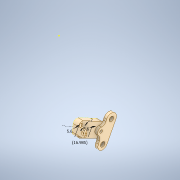
# Autodesk Inventor part: Kauri camera mount 3m bolt mount
Saved by Autodesk Inventor 2020 (Build 240168000, 168)
## iProperties
Created: 2022-04-26
Part Number: Kauri camera mount 3m bolt mount
Material: Polyethylene, High Density
Document SubType Name: Modeling
Designer: Steve3
Density: 0.952 g/cm^3
Appearance: Smooth - Off-White
Mass: 3.49117 g
Surface Area: 23.6855 cm^2
Volume: 3.6672 cm^3
Sending System: Autodesk Inventor 2020
Preprocessor: ST-DEVELOPER v18
Title: Y:\Street League\Frames\Kauri\AAA LeadFingers version 2\github files\Kauri side plate.stp
Author: Steven
Autodesk Inventor part; units mm, degrees
ref_plane "YZ Plane" through (0, 0, 0) normal (1, 0, 0) x (0, 1, 0)
ref_plane "XZ Plane" through (0, 0, 0) normal (0, 1, 0) x (-1, 0, 0)
ref_plane "XY Plane" through (0, 0, 0) normal (0, 0, 1) x (1, 0, 0)
sketch "Sketch3" plane through (0, 0, 0) normal (1, 0, 0) x (0, 1, 0)
  arc A0 (-67.955871, -10.84796) -> (-66.441009, -10.934527) centre (-66.801428, -3.943812) ccw
  line L0 (-67.955871, -10.84796) -> (-106.637607, -4.379985)
  arc A1 (-106.637607, -4.379985) -> (-109.798343, -5.963196) centre (-107.132368, -7.338906) ccw
  line L1 (-109.798343, -5.963196) -> (-127.177149, -39.641421)
  arc A2 (-127.177149, -39.641421) -> (-125.886884, -43.683106) centre (-124.511174, -41.017131) ccw
  line L2 (-125.886884, -43.683106) -> (-89.438575, -62.491345)
  arc A3 (-89.438575, -62.491345) -> (-85.311446, -54.49342) centre (-87.37501, -58.492382) ccw
  line L3 (-85.311446, -54.49342) -> (-91.002473, -51.556707)
  arc A4 (-92.937871, -45.49418) -> (-91.002473, -51.556707) centre (-88.938908, -47.557745) ccw
  line L4 (-92.937871, -45.49418) -> (-80.167513, -20.746623)
  arc A5 (-75.953198, -18.635676) -> (-80.167513, -20.746623) centre (-76.61288, -22.580903) ccw
  line L5 (-75.953198, -18.635676) -> (-69.441262, -19.724537)
  arc A6 (-69.441262, -19.724537) -> (-67.924186, -19.810989) centre (-68.286819, -12.820389) ccw
  line L6 (-67.924186, -19.810989) -> (-31.437531, -17.918268)
  arc A7 (-31.437531, -17.918268) -> (-29.900457, -17.66496) centre (-31.800164, -10.927667) ccw
  line L7 (-29.900457, -17.66496) -> (0.430435, -9.112589)
  arc A8 (1.244595, -9) -> (0.430435, -9.112589) centre (1.244595, -12) ccw
  line L8 (1.244595, -9) -> (36.324375, -9)
  arc A9 (38.324375, -11) -> (36.324375, -9) centre (36.324375, -11) ccw
  line L9 (38.324375, -11) -> (38.324375, -31.554034)
  arc A10 (38.324375, -31.554034) -> (47.324375, -31.554034) centre (42.824375, -31.554034) ccw
  line L10 (47.324375, -31.554034) -> (47.324375, -3)
  arc A11 (47.324375, -3) -> (44.324375, 0) centre (44.324375, -3) ccw
  line L11 (44.324375, 0) -> (0, 0)
  arc A12 (0, 0) -> (-0.81416, -0.112589) centre (0, -3) ccw
  line L12 (-0.81416, -0.112589) -> (-32.341858, -9.002422)
  arc A13 (-33.881146, -9.255844) -> (-32.341858, -9.002422) centre (-34.241565, -2.265129) ccw
  line L13 (-33.881146, -9.255844) -> (-66.441009, -10.934527)
  circle A14 centre (-121.30655, -39.994088) radius 1.55
  circle A15 centre (0.211343, -4.528281) radius 1.55
  circle A16 centre (42.824375, -31.554034) radius 1.55
  circle A17 centre (-105.928481, -9.742357) radius 1.55
  circle A18 centre (-101.599285, -49.7515) radius 1.55
  circle A19 centre (-31.883173, -13.503326) radius 1.55
  circle A20 centre (42.092142, -5.232233) radius 1.55
  circle A21 centre (-67.942935, -15.37073) radius 1.55
  circle A22 centre (-87.37501, -58.492382) radius 1.55
  arc A23 (-115.052095, -35.770625) -> (-113.76183, -39.81231) centre (-112.38612, -37.146335) ccw
  line L14 (-115.052095, -35.770625) -> (-105.14423, -16.570265)
  arc A24 (-100.929915, -14.459318) -> (-105.14423, -16.570265) centre (-101.589596, -18.404545) ccw
  line L15 (-100.929915, -14.459318) -> (-93.56365, -15.691031)
  arc A25 (-90.668698, -21.470538) -> (-93.56365, -15.691031) centre (-94.223331, -19.636259) ccw
  line L16 (-90.668698, -21.470538) -> (-101.165081, -41.81138)
  arc A26 (-106.553994, -43.531734) -> (-101.165081, -41.81138) centre (-104.719714, -39.9771) ccw
  line L17 (-106.553994, -43.531734) -> (-113.76183, -39.81231)
  point P0 (0, 0)
  constraints: 36 end point, 36 point on circle, 27 centre point
sketch "Sketch4" plane through (0, 0, 0) normal (1, 0, 0) x (0, 1, 0)
  circle A0 centre (-31.874031, -13.318785) radius 2.55
  circle A1 centre (-105.928481, -9.742349) radius 2.55
  circle A2 centre (-67.929027, -15.276045) radius 2.55
  arc A3 (-67.953281, -10.755052) -> (-66.596265, -10.844659) centre (-66.815732, -3.8481) ccw
  line L0 (-67.953281, -10.755052) -> (-72.057153, -10.079159)
  line L1 (-72.057153, -10.079159) -> (-106.692939, -3.305688)
  line L2 (-109.418868, -5.256805) -> (-106.692939, -3.305688)
  line L3 (-109.418868, -5.256805) -> (-109.985066, -6.360777)
  arc A4 (-109.985066, -6.360777) -> (-106.347133, -13.576326) centre (-105.536074, -8.642546) ccw
  line L4 (-106.347133, -13.576326) -> (-72.676157, -19.111461)
  line L5 (-72.676157, -19.111461) -> (-69.418112, -19.643326)
  line L6 (-69.418112, -19.643326) -> (-69.246781, -19.671535)
  arc A5 (-69.246781, -19.671535) -> (-68.163005, -19.730586) centre (-68.434471, -14.737961) ccw
  line L7 (-68.163005, -19.730586) -> (-31.193784, -17.720444)
  arc A6 (-31.193784, -17.720444) -> (-30.096328, -17.536774) centre (-31.46525, -12.727819) ccw
  line L8 (-30.096328, -17.536774) -> (-2.957928, -9.811529)
  arc A7 (-2.957928, -9.811529) -> (-2.822361, -8.911388) centre (-3.09482, -9.330633) ccw
  arc A8 (-4.999909, -2.339095) -> (-2.822361, -8.911388) centre (0.19802, -4.263787) ccw
  line L9 (-4.999909, -2.339095) -> (-5.258479, -1.511364)
  line L10 (-5.258479, -1.511364) -> (-7.95473, -1.614726)
  line L11 (-7.95473, -1.614726) -> (-29.572777, -8.030198)
  line L12 (-29.572777, -8.030198) -> (-32.007842, -8.723366)
  line L13 (-34.027372, -9.084122) -> (-32.007842, -8.723366)
  line L14 (-34.027372, -9.084122) -> (-66.596265, -10.844659)
  point P0 (0, 0)
  point P1 (-79.411985, 18.032743)
  constraints: 30 end point, 12 point on circle, 9 centre point
sketch "Sketch5" plane through (0, 0, 0) normal (1, 0, 0) x (0, 1, 0)
  line L0 (-90.668698, -21.470538) -> (-101.165081, -41.81138)
  arc A0 (-90.668698, -21.470538) -> (-93.56365, -15.691031) centre (-94.223331, -19.636259) ccw
  line L1 (-100.929915, -14.459318) -> (-93.56365, -15.691031)
  arc A1 (-100.929915, -14.459318) -> (-105.14423, -16.570265) centre (-101.589596, -18.404545) ccw
  line L2 (-115.052095, -35.770625) -> (-105.14423, -16.570265)
  arc A2 (-115.052095, -35.770625) -> (-113.76183, -39.81231) centre (-112.38612, -37.146335) ccw
  line L3 (-106.553994, -43.531734) -> (-113.76183, -39.81231)
  arc A3 (-106.553994, -43.531734) -> (-101.165081, -41.81138) centre (-104.719714, -39.9771) ccw
  line L4 (-101.253947, -41.765523) -> (-90.757564, -21.424681)
  arc A4 (-90.757564, -21.424681) -> (-93.580142, -15.789662) centre (-94.223331, -19.636259) ccw
  line L5 (-93.580142, -15.789662) -> (-100.946407, -14.557948)
  arc A5 (-100.946407, -14.557948) -> (-105.055364, -16.616122) centre (-101.589596, -18.404545) ccw
  line L6 (-105.055364, -16.616122) -> (-114.963229, -35.816482)
  arc A6 (-114.963229, -35.816482) -> (-113.715973, -39.723444) centre (-112.38612, -37.146335) ccw
  line L7 (-113.715973, -39.723444) -> (-106.508137, -43.442868)
  arc A7 (-106.508137, -43.442868) -> (-101.253947, -41.765523) centre (-104.719714, -39.9771) ccw
  point P0 (0, 0)
  dimension "d0" = 0.1
  constraints: 8 end point, 8 point on circle, 4 centre point, 7 other
  measures "d0" distance between parallel lines of L0 L4
extrude "Extrusion1" add sketch "Sketch5" along normal blind 6 contours A7 L7 A6 L6 A5 L5 A4 L4
sketch "Sketch6" plane through (0, -100.946407, -14.557948) normal (0, 0.1649204, 0.9863069) x (1, 0, 0)
  line L0 (6, 7.468532) -> (6, 0) construction
  line L1 (6, 3.734266) -> (14, 3.734266) construction
  line L2 (6, 3.734266) -> (6, 7.734266) construction
  line L3 (6, 7.734266) -> (14, 7.734266)
  line L4 (14, 7.734266) -> (14, -0.265734)
  line L5 (14, -0.265734) -> (6, -0.265734)
  line L6 (6, -0.265734) -> (6, 7.734266)
  point P0 (0, 97.163232)
  dimension "d3" = 8
  dimension "d4" = 4
  dimension "d5" = 8
  constraints: 12 end point, 2 horizontal, 2 parallel, 1 midpoint, 1 perpendicular, 1 point on line
  measures "d3" distance of L1.start L1.end
  measures "d4" distance of L1.start L2.end
  measures "d5" distance of L3.end L4.end
extrude "Extrusion2" add sketch "Sketch6" against normal blind 2
fillet "Fillet1" radius 3 2 edges at (14, -101.3734, -15.5004) (14, -93.483, -16.8198)
sketch "Sketch7" plane through (0, -101.276247, -16.530562) normal (0, -0.1649204, -0.9863069) x (-1, 0, 0)
  line L0 (-14, 4.734266) -> (-14, 2.734266)
  line L1 (-14, 2.734266) -> (-14, 4.734266) construction
  line L2 (-14, 3.734266) -> (-11.2, 3.734266) construction
  circle A0 centre (-11.2, 3.734266) radius 2.8
  circle A1 centre (-11.2, 3.734266) radius 1.5
  line L3 (-11.2, 3.734266) -> (-6, 3.734266) construction
  line L4 (-6, 7.734266) -> (-6, -0.265734) construction
  point P0 (0, 97.163232)
  dimension "d9" = 2.8
  dimension "d10" = 3
  dimension "d11" = 5.2
  constraints: 4 end point, 2 coincident, 2 midpoint, 1 centre point, 1 horizontal, 1 horizontal alignment, 2 other
  measures "d9" distance of L2.start L2.end
  measures "d10" diameter of A1
  measures "d11" distance of L3.start L3.end
fillet "Fillet2" radius 2 1 edges at (6, -97.5931, -17.1464)
fillet "Fillet3" radius 2 4 edges at (6, -93.8128, -18.7924) (6, -93.4837, -16.8243) (6, -101.7033, -17.473) (6, -101.3742, -15.5049)
extrude "Extrusion3" cut sketch "Sketch7" against normal up to surface (2 mm away) contours A1
sketch "Sketch8" plane through (6, 0, 0) normal (1, 0, 0) x (0, 0, -1)
  circle A0 centre (39.994088, -121.30655) radius 1.55 construction
  circle A1 centre (49.7515, -101.599285) radius 1.55 construction
  circle A2 centre (39.994088, -121.30655) radius 2.55
  circle A3 centre (49.7515, -101.599285) radius 2.55
  line L0 (5.963196, -109.798343) -> (39.641421, -127.177149) construction
  line L1 (43.683106, -125.886884) -> (62.491345, -89.438575) construction
  arc A4 (37.527588, -126.086359) -> (44.773897, -123.773051) centre (39.994088, -121.30655) ccw
  circle A5 centre (49.7515, -101.599285) radius 5.744834
  line L2 (44.773897, -123.773051) -> (54.856694, -104.233693)
  arc A6 (44.773897, -123.773051) -> (37.527588, -126.086359) centre (39.994088, -121.30655) ccw
  line L3 (35.21428, -118.840049) -> (44.561083, -99.137032)
  point P0 (0, 0)
  dimension "d16" = 5.1
  dimension "d17" = 5.1
  constraints: 7 point on circle, 5 centre point, 4 coincident, 4 end point, 3 tangent, 2 point on line
  measures "d16" diameter of A2
  measures "d17" diameter of A3
extrude "Extrusion4" add sketch "Sketch8" along normal blind 3
sketch "Sketch9" plane through (0, 0, 0) normal (1, 0, 0) x (0, 1, 0)
  line L0 (-98.249581, -15.008885) -> (-96.276967, -15.338725)
  line L1 (-97.263274, -15.173805) -> (-96.615466, -11.299587) construction
  line L2 (-105.928481, -9.742357) -> (-96.615466, -11.299587) construction
  point P0 (0, 0)
  dimension "d22" = 9.44231
  constraints: 4 end point, 2 perpendicular, 1 midpoint
  measures "d22" distance of L2.start L1.end
sketch "Sketch10" plane through (0, 0, 0) normal (-1, 0, 0) x (0, 0, 1)
  arc A0 (-39.723444, -113.715973) -> (-35.816482, -114.963229) centre (-37.146335, -112.38612) ccw construction
  line L0 (-16.616122, -105.055364) -> (-35.816482, -114.963229) construction
  arc A1 (-16.616122, -105.055364) -> (-14.557948, -100.946407) centre (-18.404545, -101.589596) ccw construction
  line L1 (-15.789662, -93.580142) -> (-14.557948, -100.946407) construction
  arc A2 (-15.789662, -93.580142) -> (-21.424681, -90.757564) centre (-19.636259, -94.223331) ccw construction
  line L2 (-41.765523, -101.253947) -> (-21.424681, -90.757564) construction
  arc A3 (-41.765523, -101.253947) -> (-43.442868, -106.508137) centre (-39.9771, -104.719714) ccw construction
  line L3 (-39.723444, -113.715973) -> (-43.442868, -106.508137) construction
  line L4 (-16.616122, -105.055364) -> (-35.816482, -114.963229) construction
  line L5 (-24.675821, -109.214369) -> (-31.595102, -96.005755) construction
  line L6 (-28.135461, -102.610062) -> (-45.516195, -111.714892) construction
  line L7 (-28.135461, -102.610062) -> (-2.995752, -89.440723) construction
  circle A4 centre (-28.135461, -102.610062) radius 1
  point P0 (0, 0)
  point P1 (-32.735519, -113.373375)
  dimension "d23" = 2
  constraints: 6 end point, 2 midpoint, 1 centre point, 1 coincident, 1 collinear, 1 perpendicular, 1 point on line
  measures "d23" diameter of A4
sketch "Sketch11" plane through (6, 0, 0) normal (1, 0, 0) x (0, 0, -1)
  line L0 (41.765523, -101.253947) -> (21.424681, -90.757564) construction
  arc A0 (21.424681, -90.757564) -> (16.879049, -91.465109) centre (19.636259, -94.223331) ccw construction
  line L1 (20.108555, -92.005115) -> (16.879049, -91.465109) construction
  line L2 (18.12951, -103.840797) -> (20.108555, -92.005115) construction
  line L3 (14.900003, -103.300791) -> (18.12951, -103.840797) construction
  arc A1 (14.900003, -103.300791) -> (16.616122, -105.055364) centre (18.404545, -101.589596) ccw construction
  line L4 (16.616122, -105.055364) -> (35.816482, -114.963229) construction
  line L5 (28.135461, -102.610062) -> (2.995752, -89.440723) construction
  line L6 (28.135461, -102.610062) -> (45.516195, -111.714892) construction
  line L7 (24.675821, -109.214369) -> (31.595102, -96.005755) construction
  circle A2 centre (20.522926, -98.622265) radius 1.5
  line L8 (18.12951, -103.840797) -> (20.108555, -92.005115)
  line L9 (39.129957, -99.893929) -> (32.735519, -113.373375)
  line L10 (21.851653, -99.318314) -> (33.25107, -105.289854) construction
  line L11 (39.723444, -113.715973) -> (43.442868, -106.508137) construction
  circle A3 centre (38.225648, -107.895768) radius 1.5
  circle A4 centre (38.225648, -107.895768) radius 4 construction
  line L12 (36.904981, -115.276059) -> (43.051237, -102.31978)
  arc A5 (43.051237, -102.31978) -> (41.765523, -101.253947) centre (39.9771, -104.719714) ccw
  arc A6 (35.816482, -114.963229) -> (36.904981, -115.276059) centre (37.146335, -112.38612) ccw
  point P0 (0, 0)
  dimension "d27" = 3
  dimension "d29" = 3
  dimension "d30" = 8
  constraints: 4 point on line, 2 centre point, 2 end point, 1 coincident, 1 tangent, 4 other
  measures "d29" diameter of A3
  measures "d30" diameter of A4
sketch "Sketch12" plane through (6, 0, 0) normal (1, 0, 0) x (0, 0, -1)
  circle A0 centre (38.225648, -107.895768) radius 4 construction
  circle A1 centre (38.225648, -107.895768) radius 4
  point P0 (0, 0)
  constraints: 1 centre point, 1 coincident, 1 concentric
extrude "Extrusion6" add sketch "Sketch12" along normal up to surface (3 mm away)
fillet "Fillet6" radius 5 2 edges at (7.5, -111.8854, -38.5135) (7.5, -105.5948, -41.4976)
extrude "Extrusion7" cut sketch "Sketch11" against normal through all both and the other way through all
sketch "Sketch13" plane through (0, 0, 0) normal (-1, 0, 0) x (0, 0, 1)
  circle A0 centre (-38.225648, -107.895768) radius 1.5 construction
  circle A1 centre (-38.225648, -107.895768) radius 2.8
  circle A2 centre (-20.522926, -98.622265) radius 1.5 construction
  circle A3 centre (-20.522926, -98.622265) radius 2.8
  point P0 (0, 0)
  dimension "d36" = 5.6
  dimension "d39" = 5.6
  dimension "d40" = 16.9846
  constraints: 2 centre point, 2 coincident
  measures "d36" diameter of A1
  measures "d39" diameter of A3
extrude "Extrusion8" cut sketch "Sketch13" against normal blind 3.5
body "Solid3"
